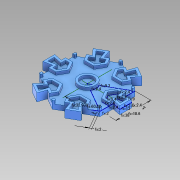
# Autodesk Inventor part: StraightRais-215
Saved by Autodesk Inventor 2021 (Build 250183000, 183)
## iProperties
Created: 2021-02-11
Part Number: StraightRais-215
Material: ABS プラスチック
Document SubType Name: Modeling
Designer: kumagai
Density: 1.06 g/cm^3
Appearance: 滑らか - 青
cp: 0.000 mm
ConnectorLength: 15.000 mm
RailWidth: 38.000 mm
JointFH: 9.500 mm
Author: kumagai
Autodesk Inventor part; units mm, degrees
ref_plane "YZ Plane" through (0, 0, 0) normal (1, 0, 0) x (0, 1, 0)
ref_plane "XZ Plane" through (0, 0, 0) normal (0, 1, 0) x (-1, 0, 0)
ref_plane "XY Plane" through (0, 0, 0) normal (0, 0, 1) x (1, 0, 0)
sketch "スケッチ1" plane through (0, 0, 0) normal (0, 1, 0) x (-1, 0, 0)
  line L0 (0, -26.6) -> (0, 26.6) projected
  line L1 (-33.6, 0) -> (5.6, 0) projected
  line L2 (-32.909, -4.7) -> (-41.909, -6.5)
  line L3 (-41.909, -6.5) -> (-41.909, 6.5)
  line L4 (-41.909, 6.5) -> (-32.909, 4.7)
  line L5 (-32.909, -19) -> (-32.909, -4.7)
  line L6 (-32.909, 4.7) -> (-32.909, 19)
  line L7 (-30.509, -1.7725) -> (-39.509, -3.5725)
  line L8 (-39.509, -3.5725) -> (-39.509, 3.5725)
  line L9 (-39.509, 3.5725) -> (-30.509, 1.7725)
  line L10 (-30.509, -6.9) -> (-30.509, -1.7725)
  line L11 (-30.509, 1.7725) -> (-30.509, 6.9)
  line L12 (0, 0) -> (-32.909, -19)
  line L13 (0, 0) -> (-32.909, 19)
  arc A0 (-8.054, 4.65) -> (-8.054, -4.65) centre (0, 0) ccw
  arc A1 (-5.9756, 3.45) -> (-5.9756, -3.45) centre (0, 0) ccw
  line L14 (-30.509, -6.9) -> (-26.3849, -6.9)
  line L15 (-26.3849, -6.9) -> (-22.4012, 0)
  line L16 (-22.4012, 0) -> (-26.3849, 6.9)
  line L17 (-26.3849, 6.9) -> (-30.509, 6.9)
  line L18 (-32.909, -9.3) -> (-24.9993, -9.3)
  line L19 (-24.9993, -9.3) -> (-19.6299, 0)
  line L20 (-19.6299, 0) -> (-24.9993, 9.3)
  line L21 (-24.9993, 9.3) -> (-32.909, 9.3)
  line L22 (-32.909, 19) -> (-27.025, 22.3971)
  line L23 (-32.909, 17) -> (-31.1769, 17)
  arc A2 (-31.1769, 17) -> (-30.3109, 17.5) centre (-31.1769, 18) ccw
  line L24 (-32.909, -17) -> (-31.1769, -17)
  arc A3 (-30.3109, -17.5) -> (-31.1769, -17) centre (-31.1769, -18) ccw
  point P0 (-19.5852, 11.3075)
  point P1 (-30.3109, -17.5)
  dimension "d2" = 9
  dimension "d3" = 13
  dimension "d5" = 9.4
  dimension "d13" = 2.4
  dimension "d14" = 2.4
  dimension "d15" = 2.4
  dimension "d24" = 2.4
  dimension "d63" = 32.909
  dimension "d64" = 38
  dimension "d66" = 2.4
  dimension "d67" = 18.6
  dimension "d68" = 2.4
  dimension "d69" = 2.4
  dimension "d70" = 2
  dimension "d78" = 60
  dimension "d79" = 2
  dimension "d80" = 1
  dimension "d81" = 9.3
  constraints: 46 end point, 11 point on line, 8 point on circle, 5 parallel, 5 symmetric about line, 4 centre point, 3 horizontal, 2 collinear, 1 coincident, 1 line through centre, 1 perpendicular, 1 tangent, 1 vertical, 6 other
  measures "d2" distance between parallel lines of L3 L5
  measures "d3" distance of L3.end L2.end
  measures "d5" distance of L4.end L2.start
  measures "d13" distance between parallel lines of L5 L10
  measures "d14" distance between parallel lines of L3 L8
  measures "d15" distance between parallel lines of L4 L9
  measures "d24" distance between parallel lines of L7 L2
  measures "d63" distance between parallel lines of L6 L0
  measures "d64" distance of L6.end L5.start
  measures "d66" radial gap between concentric circles of A1 A0
  measures "d67" distance between parallel lines of L21 L18
  measures "d68" distance between parallel lines of L21 L17
  measures "d69" distance between parallel lines of L15 L19
  measures "d70" distance from line of L6.end L20
  measures "d78" angle of L22 L13
  measures "d79" distance from line of L6.end L23
  measures "d80" radius of A2
  measures "d81" radius of A0
extrude "押し出し6" add sketch "スケッチ1" against normal blind 5.2 contours L20 L21 L6 L23 A2 L13 A0 L1 | L1 A0 L12 A3 L24 L5 L18 L19 | L19 L18 L5 L2 L3 L4 L6 L21 L20 | A0 L13 A1 L1 | L1 A1 L12 A0 | A1 L13 L1 | L1 L12 A1 | A2 L23 L6 L13 | L12 L5 L24 A3 | L7 L8 L9 L11 L17 L16 L15 L14 L10
extrude "押し出し7" add sketch "スケッチ1" along normal blind 3.2 contours L19 L18 L5 L2 L3 L4 L6 L21 L20 | A0 L13 A1 L1 | L1 A1 L12 A0 | A2 L23 L6 L13 | L12 L5 L24 A3
pattern_circular "円形状パターン1" count 6 over 360 about axis through (0, 0, 0) along (0, -1, 0) of "押し出し6", "押し出し7"
equation "\"d2\" = JointMH"
equation "\"d3\" = JointMW1 - 2 * cp"
equation "\"d5\" = JointMW2 - 2 * cp"
equation "\"d13\" = InnerWall"
equation "\"d14\" = InnerWall"
equation "\"d15\" = InnerWall"
equation "\"d24\" = InnerWall"
equation "\"Theta\" = 60deg"
equation "\"Radius\" = 38"
equation "\"CenterDist\" = 32.90897"
equation "\"JointMH\" = 9"
equation "\"JointMW1\" = 13"
equation "\"cp\" = 0"
equation "\"JointMW2\" = 9.4"
equation "\"InnerWall\" = 2.4"
